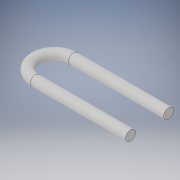
# Autodesk Inventor part: gripper_bolt
Saved by Autodesk Inventor 2019 (Build 230136000, 136)
## iProperties
Created: 2019-02-02
Part Number: gripper_bolt
Material: Generic
Document SubType Name: Modeling
Designer: suchanek
Density: 1 g/cm^3
Appearance: Default
Author: suchanek
Autodesk Inventor part; units mm, degrees
ref_plane "YZ Plane" through (0, 0, 0) normal (1, 0, 0) x (0, 1, 0)
ref_plane "XZ Plane" through (0, 0, 0) normal (0, 1, 0) x (-1, 0, 0)
ref_plane "XY Plane" through (0, 0, 0) normal (0, 0, 1) x (1, 0, 0)
sketch "Sketch1" plane through (0, 0, 0) normal (1, 0, 0) x (0, 1, 0)
  circle A0 centre (0, 0) radius 2.6
  dimension "d0" = 5.2
  constraints: 1 centre point, 1 coincident
  measures "d0" diameter of A0
sketch "Sketch2" plane through (0, 0, 0) normal (0, 1, 0) x (-1, 0, 0)
  line L0 (0, 0) -> (50, 0)
  arc A0 (50, -20) -> (50, 0) centre (50, -10) ccw
  line L1 (50, 0) -> (50, -10) construction
  line L2 (50, -20) -> (50, -10) construction
  line L3 (50, -20) -> (0, -20)
  dimension "d1" = 50
  dimension "d2" = 10
  dimension "d3" = 180
  constraints: 8 end point, 2 horizontal, 2 point on circle, 1 centre point, 1 tangent, 1 vertical alignment
  measures "d1" distance of L0.start L0.end
  measures "d2" radius of A0
  measures "d3" angle of L2 L1
sweep "Sweep1" add profiles "Sketch1" path "Sketch2"
body "Solid1"
